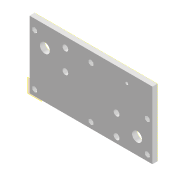
# Autodesk Inventor part: Motor mount to inside wall adapter
Saved by Autodesk Inventor 2020 (Build 240168000, 168)
## iProperties
Created: 2020-03-03
Part Number: Motor mount to inside wall adapter
Material: Generic
Document SubType Name: Modeling
Designer: ball
Density: 1 g/cm^3
Appearance: Default
Author: ball
Autodesk Inventor part; units mm, degrees
ref_plane "YZ Plane" through (0, 0, 0) normal (1, 0, 0) x (0, 1, 0)
ref_plane "XZ Plane" through (0, 0, 0) normal (0, 1, 0) x (-1, 0, 0)
ref_plane "XY Plane" through (0, 0, 0) normal (0, 0, 1) x (1, 0, 0)
ref_plane "Work Plane2" through (0, 0, 0) normal (0, 0, 1) x (1, 0, 0)
sketch "Sketch1" plane through (0, 0, 0) normal (0, 0, 1) x (1, 0, 0)
  line L0 (192, 96) -> (192, 48) construction
  line L1 (0, 96) -> (0, 48) construction
  line L2 (0, 0) -> (0, 48) construction
  line L3 (0, 0) -> (0, 96)
  line L4 (192, 96) -> (192, 0)
  circle A0 centre (184, 8) radius 2 construction
  circle A1 centre (8, 8) radius 2 construction
  circle A2 centre (8, 88) radius 2 construction
  circle A3 centre (184, 56) radius 2 construction
  arc A4 (98, 88) -> (94, 88) centre (96, 88) ccw construction
  arc A5 (94, 8) -> (98, 8) centre (96, 8) ccw construction
  circle A6 centre (184, 8) radius 2.2
  circle A7 centre (96, 8) radius 2.2
  circle A8 centre (8, 8) radius 2.2
  circle A9 centre (8, 88) radius 2.2
  circle A10 centre (96, 88) radius 2.2
  circle A11 centre (184, 56) radius 2.2
  circle A12 centre (152, 88) radius 2 construction
  circle A13 centre (152, 88) radius 2.2
  circle A14 centre (56, 88) radius 3.5 construction
  circle A15 centre (56, 56) radius 3.5 construction
  circle A16 centre (136, 8) radius 3.5 construction
  circle A17 centre (136, 40) radius 3.5 construction
  circle A18 centre (136, 8) radius 4.5
  circle A19 centre (136, 40) radius 4.5
  circle A20 centre (56, 88) radius 4.5
  circle A21 centre (56, 56) radius 4.5
  circle A22 centre (24, 72) radius 7.78 projected
  circle A23 centre (168, 24) radius 7.78 projected
  line L5 (0, 96) -> (0, 103.6708)
  line L6 (0, 103.6708) -> (192, 103.6708)
  line L7 (192, 103.6708) -> (192, 96)
  line L8 (0, 0) -> (0, -1.2954)
  line L9 (0, -1.2954) -> (192, -1.2954)
  line L10 (192, -1.2954) -> (192, 0)
  dimension "d0" = 4.4
  dimension "d1" = 4.4
  dimension "d2" = 4.4
  dimension "d3" = 4.4
  dimension "d4" = 4.4
  dimension "d5" = 4.4
  dimension "d6" = 4.4
  dimension "d7" = 9
  dimension "d8" = 9
  dimension "d9" = 9
  dimension "d10" = 9
  constraints: 16 end point, 11 centre point, 11 coincident, 3 parallel, 1 point on line
  measures "d0" diameter of A6
  measures "d1" diameter of A7
  measures "d2" diameter of A8
  measures "d3" diameter of A9
  measures "d4" diameter of A10
  measures "d5" diameter of A11
  measures "d6" diameter of A13
  measures "d7" diameter of A18
  measures "d8" diameter of A19
  measures "d9" diameter of A20
  measures "d10" diameter of A21
extrude "Extrusion1" add sketch "Sketch1" along normal blind 8
sketch "Sketch2" plane through (0, 0, 8) normal (0, 0, 1) x (1, 0, 0)
  circle A0 centre (184, 8) radius 2.2 construction
  circle A1 centre (184, 8) radius 4.115 construction
  line L0 (184, 12.115) -> (187.5637, 10.0575)
  line L1 (187.5637, 10.0575) -> (187.5637, 5.9425)
  line L2 (187.5637, 5.9425) -> (184, 3.885)
  line L3 (184, 3.885) -> (180.4363, 5.9425)
  line L4 (180.4363, 5.9425) -> (180.4363, 10.0575)
  line L5 (180.4363, 10.0575) -> (184, 12.115)
  circle A2 centre (96, 8) radius 2.2 construction
  circle A3 centre (96, 8) radius 4.115 construction
  circle A4 centre (8, 8) radius 2.2 construction
  circle A5 centre (8, 8) radius 4.115 construction
  circle A6 centre (8, 88) radius 2.2 construction
  circle A7 centre (8, 88) radius 4.115 construction
  circle A8 centre (96, 88) radius 2.2 construction
  circle A9 centre (96, 88) radius 4.115 construction
  circle A10 centre (184, 56) radius 2.2 construction
  circle A11 centre (184, 56) radius 4.115 construction
  line L6 (184, 60.115) -> (187.5637, 58.0575)
  line L7 (187.5637, 58.0575) -> (187.5637, 53.9425)
  line L8 (187.5637, 53.9425) -> (184, 51.885)
  line L9 (184, 51.885) -> (180.4363, 53.9425)
  line L10 (180.4363, 53.9425) -> (180.4363, 58.0575)
  line L11 (180.4363, 58.0575) -> (184, 60.115)
  line L12 (96, 92.115) -> (99.5637, 90.0575)
  line L13 (99.5637, 90.0575) -> (99.5637, 85.9425)
  line L14 (99.5637, 85.9425) -> (96, 83.885)
  line L15 (96, 83.885) -> (92.4363, 85.9425)
  line L16 (92.4363, 85.9425) -> (92.4363, 90.0575)
  line L17 (92.4363, 90.0575) -> (96, 92.115)
  line L18 (8, 92.115) -> (11.5637, 90.0575)
  line L19 (11.5637, 90.0575) -> (11.5637, 85.9425)
  line L20 (11.5637, 85.9425) -> (8, 83.885)
  line L21 (8, 83.885) -> (4.4363, 85.9425)
  line L22 (4.4363, 85.9425) -> (4.4363, 90.0575)
  line L23 (4.4363, 90.0575) -> (8, 92.115)
  line L24 (8, 12.115) -> (11.5637, 10.0575)
  line L25 (11.5637, 10.0575) -> (11.5637, 5.9425)
  line L26 (11.5637, 5.9425) -> (8, 3.885)
  line L27 (8, 3.885) -> (4.4363, 5.9425)
  line L28 (4.4363, 5.9425) -> (4.4363, 10.0575)
  line L29 (4.4363, 10.0575) -> (8, 12.115)
  line L30 (96, 12.115) -> (99.5637, 10.0575)
  line L31 (99.5637, 10.0575) -> (99.5637, 5.9425)
  line L32 (99.5637, 5.9425) -> (96, 3.885)
  line L33 (96, 3.885) -> (92.4363, 5.9425)
  line L34 (92.4363, 5.9425) -> (92.4363, 10.0575)
  line L35 (92.4363, 10.0575) -> (96, 12.115)
  point P0 (0, 0)
  dimension "d13" = 8.23
  dimension "d16" = 8.23
  dimension "d17" = 8.23
  dimension "d18" = 8.23
  dimension "d19" = 8.23
  dimension "d20" = 8.23
  constraints: 72 end point, 12 coincident, 6 vertical alignment, 90 other
extrude "Nut Well 4mm" cut sketch "Sketch2" against normal blind 5.5
sketch "Sketch3" plane through (0, 0, 0) normal (0, 0, -1) x (-1, 0, 0)
  circle A0 centre (-36.0247, 17.3171) radius 1.9304 construction
  circle A1 centre (-61.4247, 17.3171) radius 1.9304 construction
  circle A2 centre (-61.4247, 42.7171) radius 1.9304 construction
  circle A3 centre (-36.0247, 42.7171) radius 1.9304 construction
  circle A4 centre (-36.0247, 68.1171) radius 1.9304 construction
  circle A5 centre (-61.4247, 68.1171) radius 1.9304 construction
  circle A6 centre (-61.4247, 93.5171) radius 1.9304 construction
  circle A7 centre (-36.0247, 93.5171) radius 1.9304 construction
  circle A8 centre (-74.1247, 93.5171) radius 1.9304 construction
  circle A9 centre (-99.5247, 93.5171) radius 1.9304 construction
  circle A10 centre (-124.9247, 93.5171) radius 1.9304 construction
  circle A11 centre (-99.5247, 68.1171) radius 1.9304 construction
  circle A12 centre (-74.1247, 68.1171) radius 1.9304 construction
  circle A13 centre (-74.1247, 42.7171) radius 1.9304 construction
  circle A14 centre (-99.5247, 42.7171) radius 1.9304 construction
  circle A15 centre (-124.9247, 42.7171) radius 1.9304 construction
  line L0 (-192, -1.2954) -> (-192, 103.6708) construction
  line L1 (0, -1.2954) -> (-192, -1.2954) construction
  line L2 (0, 103.6708) -> (0, -1.2954) construction
  line L3 (-192, 103.6708) -> (0, 103.6708) construction
  circle A16 centre (-168, 24) radius 7.78 construction
  circle A17 centre (-56, 56) radius 4.5 construction
  circle A18 centre (-136, 40) radius 4.5 construction
  circle A19 centre (-184, 8) radius 2.2 construction
  circle A20 centre (-96, 8) radius 2.2 construction
  circle A21 centre (-8, 8) radius 2.2 construction
  circle A22 centre (-8, 88) radius 2.2 construction
  circle A23 centre (-96, 88) radius 2.2 construction
  circle A24 centre (-184, 56) radius 2.2 construction
  circle A25 centre (-152, 88) radius 2.2 construction
  circle A26 centre (-136, 8) radius 4.5 construction
  circle A27 centre (-56, 88) radius 4.5 construction
  circle A28 centre (-24, 72) radius 7.78 construction
  circle A29 centre (-124.9247, 68.1171) radius 1.9304 construction
  circle A30 centre (-150.3247, 68.1171) radius 1.9304 construction
  circle A31 centre (-175.7247, 68.1171) radius 1.9304 construction
  circle A32 centre (-150.3247, 42.7171) radius 1.9304 construction
  circle A33 centre (-175.7247, 42.7171) radius 1.9304 construction
  circle A34 centre (-175.7247, 17.3171) radius 1.9304 construction
  circle A35 centre (-150.3247, 17.3171) radius 1.9304 construction
  circle A36 centre (-124.9247, 17.3171) radius 1.9304 construction
  circle A37 centre (-99.5247, 17.3171) radius 1.9304 construction
  circle A38 centre (-74.1247, 17.3171) radius 1.9304 construction
  circle A39 centre (-175.7247, 93.5171) radius 1.9304 construction
  circle A40 centre (-150.3247, 93.5171) radius 1.9304 construction
  circle A41 centre (-36.0247, 17.3171) radius 1.9304
  circle A42 centre (-36.0247, 42.7171) radius 1.9304
  circle A43 centre (-36.0247, 68.1171) radius 1.9304
  circle A44 centre (-36.0247, 93.5171) radius 1.9304
  circle A45 centre (-61.4247, 68.1171) radius 1.9304
  circle A46 centre (-61.4247, 42.7171) radius 1.9304
  circle A47 centre (-61.4247, 17.3171) radius 1.9304
  circle A48 centre (-74.1247, 93.5171) radius 1.9304
  circle A49 centre (-74.1247, 17.3171) radius 1.9304
  circle A50 centre (-99.5247, 17.3171) radius 1.9304
  circle A51 centre (-124.9247, 17.3171) radius 1.9304
  circle A52 centre (-150.3247, 17.3171) radius 1.9304
  circle A53 centre (-175.7247, 17.3171) radius 1.9304
  circle A54 centre (-175.7247, 93.5171) radius 1.9304
  circle A55 centre (-124.9247, 93.5171) radius 1.9304
  circle A56 centre (-99.5247, 93.5171) radius 1.9304
  circle A57 centre (-56, 88) radius 3.5052 construction
  circle A58 centre (-61.4247, 93.5171) radius 1.9304
  point P0 (0, 0)
  dimension "SixClearanceHole" = 3.8608
  dimension "d26" = 3.8608
  dimension "d27" = 3.8608
  dimension "d28" = 3.8608
  dimension "d29" = 3.8608
  dimension "d30" = 3.8608
  dimension "d31" = 3.8608
  dimension "d32" = 3.8608
  dimension "d33" = 3.8608
  dimension "d34" = 3.8608
  dimension "d35" = 3.8608
  dimension "d36" = 3.8608
  dimension "d37" = 3.8608
  dimension "d38" = 3.8608
  dimension "d39" = 3.8608
  dimension "d40" = 3.8608
  dimension "d41" = 7.0104
  dimension "d42" = 3.8608
  constraints: 18 centre point, 18 coincident
  measures "SixClearanceHole" diameter of A41
  measures "d26" diameter of A42
  measures "d27" diameter of A43
  measures "d28" diameter of A44
  measures "d29" diameter of A45
  measures "d30" diameter of A46
  measures "d31" diameter of A47
  measures "d32" diameter of A48
  measures "d33" diameter of A49
  measures "d34" diameter of A50
  measures "d35" diameter of A51
  measures "d36" diameter of A52
  measures "d37" diameter of A53
  measures "d38" diameter of A54
  measures "d39" diameter of A55
  measures "d40" diameter of A56
  measures "d41" diameter of A57
  measures "d42" diameter of A58
extrude "Extrusion3" cut sketch "Sketch3" against normal through all
sketch "Sketch4" plane through (0, 0, 0) normal (0, 0, -1) x (-1, 0, 0)
  circle A0 centre (-36.0247, 17.3171) radius 1.9304 construction
  circle A1 centre (-36.0247, 17.3171) radius 4.6609 construction
  line L0 (-36.0247, 21.978) -> (-31.9883, 19.6475)
  line L1 (-31.9883, 19.6475) -> (-31.9883, 14.9866)
  line L2 (-31.9883, 14.9866) -> (-36.0247, 12.6562)
  line L3 (-36.0247, 12.6562) -> (-40.0612, 14.9866)
  line L4 (-40.0612, 14.9866) -> (-40.0612, 19.6475)
  line L5 (-40.0612, 19.6475) -> (-36.0247, 21.978)
  point P0 (0, 0)
  dimension "d45" = 9.3218
  constraints: 12 end point, 2 coincident, 1 vertical alignment, 15 other
extrude "Extrusion4" cut sketch "Sketch4" against normal blind 6.5024
equation "\"d26\" = SixClearanceHole"
equation "\"d27\" = SixClearanceHole"
equation "\"d28\" = SixClearanceHole"
equation "\"d29\" = SixClearanceHole"
equation "\"d30\" = SixClearanceHole"
equation "\"d31\" = SixClearanceHole"
equation "\"d32\" = SixClearanceHole"
equation "\"d33\" = SixClearanceHole"
equation "\"d34\" = SixClearanceHole"
equation "\"d35\" = SixClearanceHole"
equation "\"d36\" = SixClearanceHole"
equation "\"d37\" = SixClearanceHole"
equation "\"d38\" = SixClearanceHole"
equation "\"d39\" = SixClearanceHole"
equation "\"d40\" = SixClearanceHole"
equation "\"d42\" = SixClearanceHole"
body "Solid1"
